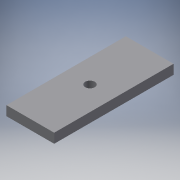
# Autodesk Inventor part: LaserMoutBottom
Saved by Autodesk Inventor 2019 (Build 230136000, 136)
## iProperties
Created: 2019-05-18
Part Number: LaserMoutBottom
Material: Generic
Document SubType Name: Modeling
Designer: Henry
Density: 1 g/cm^3
Appearance: Default
Author: Henry
Autodesk Inventor part; units mm, degrees
ref_plane "YZ Plane" through (0, 0, 0) normal (1, 0, 0) x (0, 1, 0)
ref_plane "XZ Plane" through (0, 0, 0) normal (0, 1, 0) x (-1, 0, 0)
ref_plane "XY Plane" through (0, 0, 0) normal (0, 0, 1) x (1, 0, 0)
sketch "Sketch1" plane through (0, 0, 0) normal (0, 1, 0) x (-1, 0, 0)
  line L0 (0, 0) -> (10, 0)
  line L1 (10, 0) -> (10, -12.5)
  line L2 (10, -12.5) -> (0, -12.5)
  line L3 (0, -12.5) -> (0, 0)
  dimension "d0" = 10
  dimension "d1" = 12.5
  constraints: 8 end point, 2 parallel, 1 horizontal, 1 perpendicular
  measures "d0" distance of L1.end L2.end
  measures "d1" distance of L0.end L1.end
extrude "Extrusion1" add sketch "Sketch1" along normal blind 2
sketch "Sketch2" plane through (0, 0, 0) normal (0, -1, 0) x (1, 0, 0)
  line L0 (-10, -12.5) -> (-10, 0) projected
  line L1 (-10, 0) -> (-5, 0)
  line L2 (-5, 0) -> (-5, -6.25)
  line L3 (-5, -6.25) -> (-10, -6.25)
  line L4 (-10, -6.25) -> (-10, 0)
  circle A0 centre (-5, -6.25) radius 1
  point P0 (0, 0)
  dimension "d4" = 5
  dimension "d5" = 6.25
  dimension "d6" = 2
  constraints: 8 end point, 2 parallel, 1 centre point, 1 coincident, 1 horizontal, 1 perpendicular
  measures "d4" distance of L2.end L3.end
  measures "d5" distance of L1.end L2.end
  measures "d6" diameter of A0
extrude "Extrusion2" cut sketch "Sketch2" against normal blind 2 contours A0 L2 L3 | L3 L2 A0
body "Solid1"
